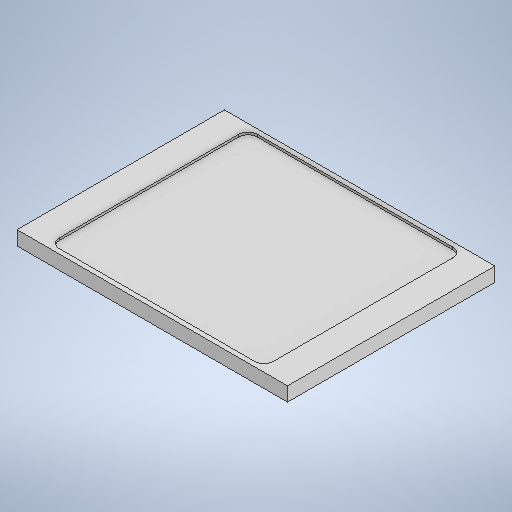
# Autodesk Inventor part: Glue Reservoir V1
Saved by Autodesk Inventor 2025 (Build 290162000, 162)
## iProperties
Created: 2026-01-29
Part Number: Glue Reservoir V1
Material: Generic
Document SubType Name: Modeling
Designer: Caleb Fangmeier
Density: 1 g/cm^3
Appearance: Default
Author: Caleb Fangmeier
Autodesk Inventor part; units mm, degrees
ref_plane "YZ Plane" through (0, 0, 0) normal (1, 0, 0) x (0, 1, 0)
ref_plane "XZ Plane" through (0, 0, 0) normal (0, 1, 0) x (-1, 0, 0)
ref_plane "XY Plane" through (0, 0, 0) normal (0, 0, 1) x (1, 0, 0)
sketch "Sketch1" plane through (0, 0, 0) normal (0, 1, 0) x (-1, 0, 0)
  line L0 (-28.75, -22.05) -> (28.75, -22.05)
  line L1 (28.75, -22.05) -> (28.75, 22.05)
  line L2 (28.75, 22.05) -> (-28.75, 22.05)
  line L3 (-28.75, 22.05) -> (-28.75, -22.05)
  line L4 (-28.75, -22.05) -> (28.75, 22.05) construction
  line L5 (28.75, -22.05) -> (-28.75, 22.05) construction
  point P0 (0, 0)
  dimension "d0" = 44.1
  dimension "d1" = 57.5
  constraints: 12 end point, 2 midpoint, 2 parallel, 1 horizontal, 1 perpendicular
  measures "d0" distance of L0.end L1.end
  measures "d1" distance of L1.end L2.end
extrude "Extrusion1" add sketch "Sketch1" along normal blind 3
sketch "Sketch2" plane through (0, 3, 0) normal (0, 1, 0) x (1, 0, 0)
  line L0 (20.75, 21.05) -> (-20.75, 21.05)
  line L1 (-22.75, 19.05) -> (-22.75, -19.05)
  line L2 (-20.75, -21.05) -> (20.75, -21.05)
  line L3 (22.75, -19.05) -> (22.75, 19.05)
  line L4 (22.75, 21.05) -> (-22.75, -21.05) construction
  line L5 (-22.75, 21.05) -> (22.75, -21.05) construction
  line L6 (-28.75, 22.05) -> (-28.75, -22.05) projected
  line L7 (-28.75, -22.05) -> (28.75, -22.05) projected
  arc A0 (-22.75, -19.05) -> (-20.75, -21.05) centre (-20.75, -19.05) ccw
  arc A1 (-20.75, 21.05) -> (-22.75, 19.05) centre (-20.75, 19.05) ccw
  arc A2 (22.75, 19.05) -> (20.75, 21.05) centre (20.75, 19.05) ccw
  arc A3 (20.75, -21.05) -> (22.75, -19.05) centre (20.75, -19.05) ccw
  point P0 (0, 0)
  dimension "d4" = 6
  dimension "d5" = 1
  dimension "d6" = 2
  constraints: 12 end point, 8 point on circle, 8 point on line, 8 tangent, 4 centre point, 3 equal radius, 2 midpoint, 2 parallel, 1 horizontal, 1 perpendicular
  measures "d4" distance between parallel lines of L6 L1
  measures "d5" distance between parallel lines of L7 L2
  measures "d6" radius of A0
extrude "Extrusion2" cut sketch "Sketch2" against normal blind 0.5
body "Solid1"
